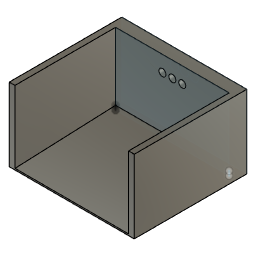
robot scooper 1 v3 (Autodesk Fusion 360 design; units mm, degrees)
Autodesk Fusion 360 part; units mm, degrees
sketch "Sketch1" plane through (0, 0, 0) normal (0, 0, 1) x (1, 0, 0)
  line L0 (0, 0) -> (81, 0)
  line L1 (81, 0) -> (81, 71)
  line L2 (81, 71) -> (0, 71)
  line L3 (0, 71) -> (0, 0)
  dimension "d1" = 81
  dimension "d2" = 71
  constraint horizontal L0
  constraint vertical L1
  constraint horizontal L2
  constraint vertical L3
  constraint coincident L0.start L3.end
  measures "d1" distance of L0.start L0.end
  measures "d2" distance of L0.start L2.end
extrude "Extrude1" add sketch "Sketch1" along normal blind 1
sketch "Sketch2" plane through (0, 0, 0) normal (1, 0, 0) x (0, 1, 0)
sketch "Sketch3" plane through (0, 0, 1) normal (0, 0, 1) x (-1, 0, 0)
  line L0 (0, -71) -> (0, 0)
  line L1 (0, 0) -> (-81, 0)
  line L2 (-81, 0) -> (-81, -71)
  line L3 (-81, -71) -> (0, -71)
  line L4 (0, -71) -> (-1, -71)
  line L5 (-1, -71) -> (-1, 0)
  line L6 (-1, 0) -> (0, 0)
  line L7 (0, 0) -> (0, -71)
  line L8 (-81, -71) -> (-80, -71)
  line L9 (-80, -71) -> (-80, 0)
  line L10 (-80, 0) -> (-81, 0)
  line L11 (-81, 0) -> (-81, -71)
  line L12 (-1, -71) -> (-80, -71)
  line L13 (-80, -71) -> (-80, -70)
  line L14 (-80, -70) -> (-1, -70)
  line L15 (-1, -70) -> (-1, -71)
  dimension "d5" = 1
  dimension "d6" = 1
  dimension "d7" = 1
  constraint horizontal L4
  constraint vertical L5
  constraint horizontal L6
  constraint vertical L7
  constraint coincident L0.start L3.end
  constraint horizontal L8
  constraint vertical L9
  constraint horizontal L10
  constraint vertical L11
  constraint coincident L2.end L3.start
  constraint horizontal L12
  constraint vertical L13
  constraint horizontal L14
  constraint vertical L15
  constraint coincident L9 L13.end
  measures "d5" distance of L0.start L4.end
  measures "d6" distance of L2.end L8.end
  measures "d7" distance of L4.end L14.end
extrude "Extrude2" add sketch "Sketch3" along normal blind 50 contours L3 L5 L9 L12 L13 L14 L15
sketch "Sketch4" plane through (0, 0, 1) normal (0, 0, 1) x (-1, 0, 0)
  line L0 (-80, -71) -> (-80, -70)
  line L1 (-80, -70) -> (-1, -70)
  line L2 (-1, -70) -> (-1, -71)
  line L3 (-1, -71) -> (0, -71)
  line L4 (0, -71) -> (0, 0)
  line L5 (0, 0) -> (-81, 0)
  line L6 (-81, 0) -> (-81, -71)
  line L7 (-81, -71) -> (-80, -71)
  line L8 (0, 0) -> (-1, 0)
  line L9 (-1, 0) -> (-1, -71)
  line L10 (-1, -71) -> (0, -71)
  line L11 (0, -71) -> (0, 0)
  dimension "d10" = 1
  dimension "d11" = 71
  constraint horizontal L8
  constraint vertical L9
  constraint horizontal L10
  constraint vertical L11
  constraint coincident L4.end L5.start
  measures "d10" distance of L4.end L8.end
  measures "d11" distance of L4.end L3.end
extrude "Extrude3" add sketch "Sketch4" along normal blind 50 contours L2 L3 L4 L5 L8 L9 L10 L11
sketch "Sketch5" plane through (0, 0, 1) normal (0, 0, 1) x (-1, 0, 0)
  line L0 (-1, -70) -> (-1, 0)
  line L1 (-1, 0) -> (-81, 0)
  line L2 (-81, 0) -> (-81, -71)
  line L3 (-81, -71) -> (-80, -71)
  line L4 (-80, -71) -> (-80, -70)
  line L5 (-80, -70) -> (-1, -70)
  line L6 (-81, 0) -> (-80, 0)
  line L7 (-80, 0) -> (-80, -71)
  line L8 (-80, -71) -> (-81, -71)
  line L9 (-81, -71) -> (-81, 0)
  dimension "d14" = 71
  constraint horizontal L6
  constraint vertical L7
  constraint horizontal L8
  constraint vertical L9
  constraint coincident L1.end L2.start
  measures "d14" distance of L1.end L2.end
extrude "Extrude4" add sketch "Sketch5" along normal blind 50 contours L1 L2 L3 L4 L6 L7 L8 L9
sketch "Sketch6" plane through (0, 70, 0) normal (0, -1, 0) x (1, 0, 0)
  line L0 (1, 1) -> (80, 1)
  line L1 (80, 1) -> (80, 51)
  line L2 (80, 51) -> (1, 51)
  line L3 (1, 51) -> (1, 1)
  line L4 (80, 1) -> (80, 4)
  line L5 (1, 4) -> (1, 1)
  dimension "d17" = 79
  dimension "d18" = 3
  constraint vertical L4
  constraint vertical L5
  constraint coincident L0.start L3.end
  measures "d17" distance of L0.start L0.end
  measures "d18" distance of L0.start L5.start
sketch "Sketch7" plane through (0, 70, 0) normal (0, -1, 0) x (1, 0, 0)
extrude "Extrude5" cut 1 faces at (27.3333, 46.6667, 1) along direction (0, 0, -1) blind 1
sketch "Sketch8" plane through (0, 0, 0) normal (0, 1, 0) x (1, 0, 0)
sketch "Sketch9" plane through (1, 0, 0) normal (1, 0, 0) x (0, 1, 0)
  line L0 (70, 0) -> (70, 51)
  line L1 (70, 51) -> (0, 51)
  line L2 (0, 51) -> (0, 0)
  line L3 (0, 0) -> (70, 0)
  line L4 (0, 0) -> (70, 0)
  line L5 (70, 0) -> (70, 1)
  line L6 (70, 1) -> (0, 1)
  line L7 (0, 1) -> (0, 0)
  dimension "d21" = 70
  dimension "d22" = 1
  constraint horizontal L4
  constraint vertical L5
  constraint horizontal L6
  constraint vertical L7
  constraint coincident L2.end L3.start
  measures "d21" distance of L2.end L0.start
  measures "d22" distance of L2.end L6.end
extrude "Extrude6" add sketch "Sketch9" along normal blind 79 contours L0 L2 L3 L4 L5 L6 L7
sketch "Sketch10" plane through (80, 0, 0) normal (-1, 0, 0) x (0, -1, 0)
  line L0 (-70, 1) -> (0, 1)
  line L1 (0, 1) -> (0, 51)
  line L2 (0, 51) -> (-70, 51)
  line L3 (-70, 51) -> (-70, 1)
  line L4 (-70, 1) -> (-70, 4)
  line L5 (-70, 4) -> (0, 1)
  line L6 (-70, 1) -> (-70, 4)
  constraint coincident L0.start L3.end
  constraint coincident L3 L4.end
  constraint coincident L0.end L1.start
extrude "Extrude7" add sketch "Sketch10" along normal blind 79 contours L0 L3 L4 L5 L6
sketch "Sketch11" plane through (0, 0, 0) normal (0, 0, 1) x (1, 0, 0)
  line L0 (0, 0) -> (-3, 0)
  line L1 (-3, 0) -> (-3, 74)
  line L2 (-3, 74) -> (0, 74)
  line L3 (0, 74) -> (0, 0)
  dimension "d27" = 3
  dimension "d28" = 74
  constraint horizontal L0
  constraint vertical L1
  constraint horizontal L2
  constraint vertical L3
  constraint coincident L0.start L3.end
  measures "d27" distance of L0.start L0.end
  measures "d28" distance of L0.start L2.end
extrude "Extrude8" add sketch "Sketch11" along normal blind 51
sketch "Sketch12" plane through (0, 0, 0) normal (1, 0, 0) x (0, 1, 0)
  line L0 (71, 51) -> (71, 0)
  line L1 (71, 0) -> (74, 0)
  line L2 (74, 0) -> (74, 51)
  line L3 (74, 51) -> (71, 51)
  line L4 (74, 51) -> (71, 51)
  line L5 (71, 51) -> (71, 0)
  line L6 (71, 0) -> (74, 0)
  line L7 (74, 0) -> (74, 51)
  constraint horizontal L4
  constraint vertical L5
  constraint horizontal L6
  constraint vertical L7
  constraint coincident L0.end L1.start
  constraint coincident L2.end L3.start
extrude "Extrude9" add sketch "Sketch12" along normal blind 84
sketch "Sketch13" plane through (0, 71, 0) normal (0, -1, 0) x (1, 0, 0)
  line L0 (81, 51) -> (81, 0)
  line L1 (81, 0) -> (84, 0)
  line L2 (84, 0) -> (84, 51)
  line L3 (84, 51) -> (81, 51)
  line L4 (81, 51) -> (84, 51)
  line L5 (84, 51) -> (84, 0)
  line L6 (84, 0) -> (81, 0)
  line L7 (81, 0) -> (81, 51)
  constraint horizontal L4
  constraint vertical L5
  constraint horizontal L6
  constraint vertical L7
  constraint coincident L1.end L2.start
  constraint coincident L0.start L3.end
extrude "Extrude10" add sketch "Sketch13" along normal blind 71
sketch "Sketch14" plane through (0, 74, 0) normal (0, 1, 0) x (-1, 0, 0)
  line L0 (-84, 0) -> (3, 0)
  line L1 (3, 0) -> (3, 51)
  line L2 (3, 51) -> (-84, 51)
  line L3 (-84, 51) -> (-84, 0)
extrude "Extrude11" add sketch "Sketch14" along normal blind 4.3
sketch "Sketch15" plane through (0, 78.3, 0) normal (0, 1, 0) x (-1, 0, 0)
  line L0 (-84, 51) -> (-84, 0)
  line L1 (-84, 0) -> (3, 0)
  line L2 (3, 0) -> (3, 51)
  line L3 (3, 51) -> (-84, 51)
  line L4 (-79, 40) -> (-84, 40)
  circle A0 centre (-40.5, 40) radius 2.95
  dimension "d37" = 43.5
  dimension "d38" = 5.9
  constraint coincident L0 L4.end
  constraint perpendicular L0 L4
  measures "d37" distance of L4.end A0.centre
  measures "d38" diameter of A0
extrude "Extrude12" cut sketch "Sketch15" against normal blind 0.8 contours A0
sketch "Sketch16" plane through (0, 77.5, 0) normal (0, 1, 0) x (-1, 0, 0)
  circle A0 centre (-40.5, 40) radius 2.95
  circle A1 centre (-40.5, 40) radius 2.45
  dimension "d41" = 4.9
  constraint concentric A0 A1
  measures "d41" diameter of A1
extrude "Extrude13" cut sketch "Sketch16" against normal blind 10 contours A1
sketch "Sketch17" plane through (0, 78.3, 0) normal (0, 1, 0) x (-1, 0, 0)
  circle A0 centre (-40.5, 40) radius 2.95
  line L0 (-84, 51) -> (-84, 0)
  line L1 (-84, 0) -> (3, 0)
  line L2 (3, 0) -> (3, 51)
  line L3 (3, 51) -> (-84, 51)
  line L4 (-40.5, 42.95) -> (-40.5, 40)
  line L5 (-40.5, 40) -> (-37.55, 40)
  line L6 (-37.55, 40) -> (-36.55, 40)
  line L7 (-36.55, 40) -> (-33.6, 40)
  circle A1 centre (-33.6, 40) radius 2.95
  dimension "d44" = 2.95
  dimension "d45" = 1
  dimension "d46" = 2.95
  dimension "d47" = 5.9
  constraint coincident A0 L4.start
  constraint coincident A0.centre L4.end
  constraint vertical L4
  constraint perpendicular L4 L5
  constraint parallel L5 L6
  constraint perpendicular L4 L7
  constraint coincident L7.end A1.centre
  measures "d44" distance of A0.centre L5.end
  measures "d45" distance of L5.end L6.end
  measures "d46" distance of L6.end L7.end
  measures "d47" diameter of A1
extrude "Extrude14" cut sketch "Sketch17" against normal blind 0.8 contours A1
sketch "Sketch18" plane through (0, 77.5, 0) normal (0, 1, 0) x (-1, 0, 0)
  circle A0 centre (-33.6, 40) radius 2.95
  circle A1 centre (-33.6, 40) radius 2.45
  dimension "d50" = 4.9
  constraint concentric A0 A1
  measures "d50" diameter of A1
extrude "Extrude15" cut sketch "Sketch18" against normal blind 10 contours A1
sketch "Sketch19" plane through (0, 78.3, 0) normal (0, 1, 0) x (-1, 0, 0)
  circle A0 centre (-33.6, 40) radius 2.95
  circle A1 centre (-40.5, 40) radius 2.95
  line L0 (-84, 51) -> (-84, 0)
  line L1 (-84, 0) -> (3, 0)
  line L2 (3, 0) -> (3, 51)
  line L3 (3, 51) -> (-84, 51)
  line L4 (-40.5, 40) -> (-43.45, 40)
  line L5 (-43.45, 40) -> (-44.45, 40)
  line L6 (-44.45, 40) -> (-47.4, 40)
  circle A2 centre (-47.4, 40) radius 2.95
  dimension "d53" = 2.95
  dimension "d54" = 1
  dimension "d55" = 2.95
  dimension "d57" = 5.9
  constraint coincident A1.centre L4.start
  constraint horizontal L4
  constraint horizontal L5
  constraint parallel L5 L6
  measures "d53" distance of A1.centre L4.end
  measures "d54" distance of L4.end L5.end
  measures "d55" distance of L5.end L6.end
  measures "d57" diameter of A2
extrude "Extrude16" cut sketch "Sketch19" against normal blind 0.8 contours A2
sketch "Sketch20" plane through (0, 77.5, 0) normal (0, 1, 0) x (-1, 0, 0)
  circle A0 centre (-47.4, 40) radius 2.95
  circle A1 centre (-47.4, 40) radius 2.45
  dimension "d60" = 4.9
  constraint concentric A0 A1
  measures "d60" diameter of A1
extrude "Extrude17" cut sketch "Sketch20" against normal blind 10 contours A1
sketch "Sketch21" plane through (0, 78.3, 0) normal (0, 1, 0) x (-1, 0, 0)
  circle A0 centre (-47.4, 40) radius 2.95
  circle A1 centre (-33.6, 40) radius 2.95
  circle A2 centre (-40.5, 40) radius 2.95
  line L0 (-84, 51) -> (-84, 0)
  line L1 (-84, 0) -> (3, 0)
  line L2 (3, 0) -> (3, 51)
  line L3 (3, 51) -> (-84, 51)
equation "d37 = ( 87 / 2 ) * 1 mm"
equation "d44 = ( 5.9 / 2 ) * 1 mm"
equation "d46 = ( 5.9 / 2 ) * 1 mm"
equation "d53 = ( 5.9 / 2 ) * 1 mm"
equation "d55 = ( 5.9 / 2 ) * 1 mm"
